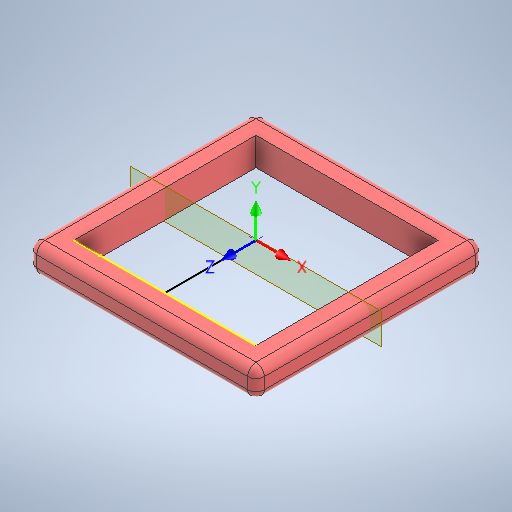
# Autodesk Inventor part: 2025 Bumper Fabric
Saved by Autodesk Inventor 2025 (Build 290162000, 162)
## iProperties
Created: 2025-01-15
Part Number: 2025 Bumper Fabric
Material: Generic
Document SubType Name: Modeling
Designer: Test
Density: 1 g/cm^3
Appearance: Default
Author: Test
Autodesk Inventor part; units mm, degrees
ref_plane "YZ Plane" through (0, 0, 0) normal (1, 0, 0) x (0, 1, 0)
ref_plane "XZ Plane" through (0, 0, 0) normal (0, 1, 0) x (-1, 0, 0)
ref_plane "XY Plane" through (0, 0, 0) normal (0, 0, 1) x (1, 0, 0)
sketch "Sketch1" plane through (0, 0, 0) normal (0, 0, 1) x (1, 0, 0)
  line L0 (-206.4033, 0) -> (746.0967, 0)
  line L1 (746.0967, 0) -> (746.0967, 117.475)
  line L2 (746.0967, 117.475) -> (-206.4033, 117.475)
  line L3 (-206.4033, 117.475) -> (-206.4033, 0)
  point P0 (0, 0)
  dimension "d0" = 952.5
  dimension "d1" = 117.475
  constraints: 8 end point, 2 perpendicular, 1 horizontal, 1 vertical
  measures "d0" distance of L0.start L0.end
  measures "d1" distance of L0.end L1.end
extrude "Extrusion1" add sketch "Sketch1" along normal blind 95.25
sketch "Sketch3" plane through (-206.4033, 117.475, 0) normal (0, 1, 0) x (1, 0, 0)
  line L0 (952.5, 0) -> (0, 0) projected
  line L1 (0, 0) -> (95.25, 0)
  line L2 (952.5, -95.25) -> (0, -95.25) projected
  line L3 (95.25, 0) -> (0, -95.25)
  line L4 (952.5, 0) -> (857.25, 0)
  line L5 (857.25, 0) -> (952.5, -95.25)
  line L6 (0, -95.25) -> (0, 0)
  line L7 (0, 0) -> (95.25, 0)
  line L8 (857.25, 0) -> (952.5, 0)
  line L9 (952.5, 0) -> (952.5, -95.25)
  line L10 (95.25, 0) -> (857.25, 0)
  point P0 (206.4033, 0)
  dimension "d6" = 95.25
  dimension "d7" = 95.25
  constraints: 18 end point, 3 collinear, 2 point on line, 1 perpendicular
  measures "d6" distance of L0.end L1.end
  measures "d7" distance of L0.start L4.end
extrude "Extrusion2" cut sketch "Sketch3" against normal through all contours L9 L5 L0 | L3 L6 L0
fillet "Fillet1" radius 34.925 2 edges at (269.8467, 0, 95.25) (269.8467, 117.475, 95.25)
shell "Shell1" [suppressed]
sketch "Sketch4" plane through (-111.1533, 117.475, 0) normal (0, 1, 0) x (1, 0, 0)
  line L0 (762, 0) -> (0, 0) projected
  line L1 (381, 0) -> (381, 381)
  point P0 (111.1533, 0)
  constraints: 2 end point, 1 coincident, 1 midpoint, 1 vertical
ref_plane "Work Plane1" through (269.8467, 107.475, -381) normal (0, 0, -1) x (0, 1, 0)
pattern_circular "Circular Pattern1" count 4 over 360 about axis through (269.8467, 107.475, -381) along (0, 1, 0)
fillet "Fillet3" radius 34.925 12 edges at (-196.174, 107.2457, -847.0207) (-196.174, 10.2293, -847.0207) (-206.4033, 58.7375, -857.25) (746.0967, 58.7375, -857.25) (735.8674, 10.2293, -847.0207) (735.8674, 107.2457, -847.0207) (735.8674, 107.2457, 85.0207) (735.8674, 10.2293, 85.0207) (746.0967, 58.7375, 95.25) (-196.174, 10.2293, 85.0207) (-196.174, 107.2457, 85.0207) (-206.4033, 58.7375, 95.25)
body "Solid1"
